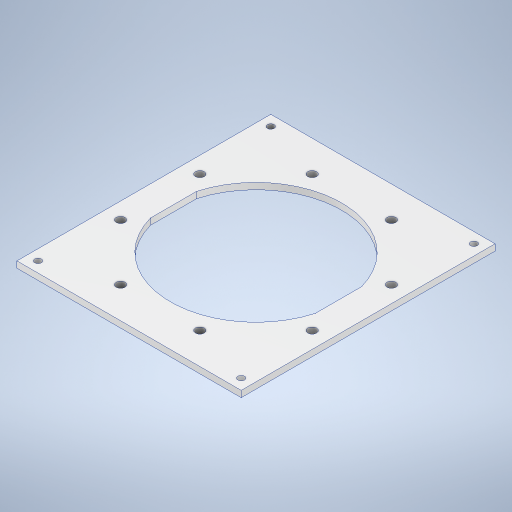
# Autodesk Inventor part: link2_plate2
Saved by Autodesk Inventor 2024 (Build 280153000, 153)
## iProperties
Created: 2024-12-13
Part Number: link2_plate2
Material: アルミニウム 6061
Document SubType Name: Sheet Metal
Designer: hirek
Density: 2.7 g/cm^3
Sheet Metal Rule: Default_mm
Appearance: アルミニウム - フラット
Author: hirek
Autodesk Inventor part; units mm, degrees
ref_plane "YZ Plane" through (0, 0, 0) normal (1, 0, 0) x (0, 1, 0)
ref_plane "XZ Plane" through (0, 0, 0) normal (0, 1, 0) x (-1, 0, 0)
ref_plane "XY Plane" through (0, 0, 0) normal (0, 0, 1) x (1, 0, 0)
sketch "スケッチ1" plane through (0, 0, 0) normal (0, 1, 0) x (-1, 0, 0)
  line L0 (0, 0) -> (106, 0)
  line L1 (106, 0) -> (106, -120)
  line L2 (106, -120) -> (0, -120)
  line L3 (0, -120) -> (0, 0)
  dimension "d0" = 106
  dimension "d1" = 120
  constraints: 8 end point, 2 parallel, 1 horizontal, 1 perpendicular
  measures "d0" distance of L1.end L2.end
  measures "d1" distance of L0.end L1.end
extrude "押し出し1" add sketch "スケッチ1" along normal blind 3
sketch "スケッチ2" plane through (0, 3, 0) normal (0, 1, 0) x (1, 0, 0)
  line L0 (-106, 120) -> (-106, 0) projected
  line L1 (0, 120) -> (-106, 120) projected
  line L2 (-106, 0) -> (0, 120)
  circle A0 centre (-53, 60) radius 49
  line L3 (-106, 60) -> (0, 60)
  line L4 (0, 0) -> (0, 120) projected
  line L5 (-53, 60) -> (-7.7299, 78.7515)
  point P0 (-34.2485, 105.2701)
  point P1 (-71.7515, 105.2701)
  point P2 (-98.2701, 78.7515)
  point P3 (-98.2701, 41.2485)
  point P4 (-71.7515, 14.7299)
  point P5 (-34.2485, 14.7299)
  point P6 (-7.7299, 41.2485)
  dimension "d4" = 98
  dimension "d5" = 22.5
  dimension "d8" = 360
  constraints: 6 end point, 3 midpoint, 2 coincident, 18 other
  measures "d5" angle of L5 L3
hole "穴1" at (-7.7299, 3, -78.7515) at (-34.2485, 3, -105.2701) at (-71.7515, 3, -105.2701) at (-98.2701, 3, -78.7515) at (-98.2701, 3, -41.2485) at (-71.7515, 3, -14.7299) at (-34.2485, 3, -14.7299) at (-7.7299, 3, -41.2485) direction (0, -1, 0) diameter 4.2 end through all
sketch "スケッチ3" plane through (0, 3, 0) normal (0, 1, 0) x (1, 0, 0)
  line L0 (-106, 120) -> (-106, 0) projected
  line L1 (0, 120) -> (-106, 120) projected
  line L2 (-106, 0) -> (0, 120)
  circle A0 centre (-53, 60) radius 40.5
  line L3 (-106, 0) -> (0, 0) projected
  line L4 (-92, 0) -> (-92, 120)
  line L5 (-14, 0) -> (-14, 120)
  point P0 (-14, 60)
  point P1 (-92, 70.9202)
  point P2 (-92, 49.0798)
  point P3 (-14, 49.0798)
  point P4 (-14, 70.9202)
  dimension "d17" = 81
  dimension "d20" = 39
  dimension "d21" = 39
  constraints: 6 end point, 4 point on line, 2 midpoint, 2 perpendicular, 1 centre point
  measures "d17" diameter of A0
  measures "d20" distance from line of L4 A0.centre
  measures "d21" distance of point (-14, 60) A0.centre
extrude "押し出し2" cut sketch "スケッチ3" against normal blind 3 contours A0 L2 L4 | L2 A0 L5 picked at (-69.0671, 72.6536) picked at (-40, 56.3599)
sketch "スケッチ4" plane through (0, 3, 0) normal (0, 1, 0) x (1, 0, 0)
  line L0 (-106, 120) -> (-106, 0) projected
  line L1 (-106, 5) -> (0, 5)
  line L2 (0, 0) -> (0, 120) projected
  line L3 (-120, 115) -> (0, 115)
  line L4 (-106, 0) -> (0, 0) projected
  line L5 (0, 120) -> (-106, 120) projected
  line L6 (-106, 0) -> (0, 0) projected
  line L7 (-101, 0) -> (-101, 120)
  line L8 (-5, 120) -> (-5, 0)
  point P0 (-101, 5)
  point P1 (-5, 5)
  point P2 (-5, 115)
  point P3 (-101, 115)
  dimension "d22" = 5
  dimension "d23" = 5
  dimension "d24" = 5
  dimension "d25" = 5
  constraints: 14 point on line, 8 end point, 2 horizontal, 2 perpendicular
  measures "d22" distance between parallel lines of L1 L4
  measures "d23" distance between parallel lines of L5 L3
  measures "d24" distance between parallel lines of L0 L7
  measures "d25" distance between parallel lines of L2 L8
hole "穴2" at (-101, 3, -5) at (-5, 3, -5) at (-5, 3, -115) at (-101, 3, -115) direction (0, -1, 0) diameter 3.2 end through all
equation "\"d15\" = Thickness"
equation "\"BendRadius\" = Thickness"
equation "\"BendReliefWidth\" = Thickness"
equation "\"BendReliefDepth\" = 0.5 * Thickness"
equation "\"CornerReliefSize\" = 4 * Thickness"
equation "\"MinimumRemnant\" = 2 * Thickness"
equation "\"TransitionRadius\" = BendRadius"
equation "\"JacobiRadiusSize\" = BendRadius"
equation "\"GapSize\" = Thickness"
equation "\"Thickness\" = 0.5"
